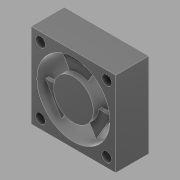
# Autodesk Inventor part: maly_wentylator
Saved by Autodesk Inventor 2021 (Build 250183000, 183)
## iProperties
Created: 2022-10-18
Part Number: maly_wentylator
Material: Generic
Document SubType Name: Modeling
Designer: agnpi
Density: 1 g/cm^3
Appearance: Smooth - Black
Author: agnpi
Autodesk Inventor part; units mm, degrees
ref_plane "YZ Plane" through (0, 0, 0) normal (1, 0, 0) x (0, 1, 0)
ref_plane "XZ Plane" through (0, 0, 0) normal (0, 1, 0) x (-1, 0, 0)
sketch "Sketch1" plane through (0, 0, 0) normal (0, 0, 1) x (1, 0, 0)
  line L0 (0, -17.85) -> (0, 17.85) construction
  line L1 (-17.85, 0) -> (17.85, 0) construction
  line L2 (-12.75, 12.75) -> (12.75, 12.75)
  line L3 (12.75, 12.75) -> (12.75, -12.75)
  line L4 (12.75, -12.75) -> (-12.75, -12.75)
  line L5 (-12.75, -12.75) -> (-12.75, 12.75)
  line L6 (-12.75, 12.75) -> (12.75, -12.75) construction
  line L7 (12.75, 12.75) -> (-12.75, -12.75) construction
  circle A0 centre (-10, -10) radius 1.5
  circle A1 centre (10, -10) radius 1.5
  circle A2 centre (-10, 10) radius 1.5
  circle A3 centre (10, 10) radius 1.5
  circle A4 centre (0, 0) radius 6
  circle A5 centre (0, 0) radius 11
  dimension "d0" = 25.5
  dimension "d1" = 25.5
  dimension "d2" = 3
  dimension "d3" = 3
  dimension "d4" = 20
  dimension "d5" = 2.75
  dimension "d7" = 2.75
  dimension "d8" = 2.75
  dimension "d9" = 12
  dimension "d10" = 22
  constraints: 12 end point, 6 centre point, 2 coincident, 2 midpoint, 2 parallel, 2 symmetric about line, 1 horizontal, 1 perpendicular, 2 other
  measures "d0" distance of L3.end L4.end
  measures "d1" distance of L2.end L3.end
  measures "d2" diameter of A0
  measures "d3" diameter of A1
  measures "d4" distance of A1.centre A0.centre
  measures "d5" distance from line of L5 A0.centre
  measures "d7" distance from line of L3 A1.centre
  measures "d8" distance from line of L4 A0.centre
  measures "d9" diameter of A4
  measures "d10" diameter of A5
extrude "Extrusion1" add sketch "Sketch1" along normal blind 10
extrude "Extrusion2" add sketch "Sketch1" along normal blind 1 contours A5
sketch "Sketch3" plane through (0, 0, 0) normal (0, 0, -1) x (-1, 0, 0)
  circle A0 centre (0, 0) radius 6 projected
  line L0 (-5.4158, 2.5824) -> (-9.7489, 5.095)
  circle A1 centre (0, 0) radius 11 projected
  line L1 (-4.9551, 3.3833) -> (-9.2869, 5.8953)
  line L2 (0.4715, -5.9814) -> (0.462, -10.9903)
  line L3 (-0.4525, -5.9829) -> (-0.462, -10.9903)
  line L4 (4.9443, 3.399) -> (9.2869, 5.8953)
  line L5 (5.4076, 2.5996) -> (9.7489, 5.095)
  dimension "d17" = 0.924
  dimension "d18" = 0.924
  dimension "d21" = 360
  dimension "d23" = 120
  dimension "d24" = 0.924
  constraints: 12 end point, 4 point on circle, 19 other
  measures "d17" distance of L0.start L1.start
  measures "d18" distance of L1.end L0.end
  measures "d23" angle of L3 L0
  measures "d24" distance of L2.end L3.end
extrude "Extrusion3" cut sketch "Sketch3" against normal blind 1 contours A0 L5 A1 L2 | A0 L1 A1 L4 | L3 A1 L0 A0
ref_plane "Work Plane1" through (0, 0, 8.4) normal (0, 0, 1) x (1, 0, 0)
sketch "Sketch4" plane through (0, 0, 8.4) normal (0, 0, 1) x (1, 0, 0)
  circle A0 centre (0, 0) radius 6 projected
  line L0 (-2.75, 5.3327) -> (-4.75, 8.7968)
  line L1 (-4.75, 8.7968) -> (4.75, 8.7968)
  line L2 (4.75, 8.7968) -> (2.75, 5.3327)
  line L3 (-12.75, 12.75) -> (-12.75, -12.75) projected
  line L4 (12.75, -12.75) -> (12.75, 12.75) projected
  line L5 (-3.2432, -5.0479) -> (-5.2432, -8.512)
  line L6 (-5.2432, -8.512) -> (-9.9932, -0.2848)
  line L7 (-9.9932, -0.2848) -> (-5.9932, -0.2848)
  line L8 (5.9932, -0.2848) -> (9.9932, -0.2848)
  line L9 (9.9932, -0.2848) -> (5.2432, -8.512)
  line L10 (5.2432, -8.512) -> (3.2432, -5.0479)
  dimension "d28" = 8
  dimension "d29" = 8
  dimension "d30" = 10
  dimension "d31" = 60
  dimension "d32" = 60
  dimension "d35" = 360
  constraints: 18 end point, 2 point on circle, 1 horizontal, 22 other
  measures "d28" distance from line of L3 L0.end
  measures "d29" distance from line of L4 L1.end
  measures "d30" distance from line of L4 L2.end
  measures "d31" angle of L0 L1
  measures "d32" angle of L2 L1
extrude "Extrusion4" add sketch "Sketch4" against normal blind 1 contours A0 L0 L1 L2 | L8 L9 L10 A0 | A0 L5 L6 L7
body "Solid1"
